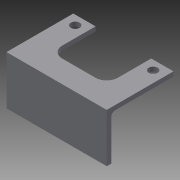
# Autodesk Inventor part: stpper holder
Saved by Autodesk Inventor 2015 (Build 190159000, 159)
## iProperties
Created: 2016-05-27
Part Number: stpper holder
Material: Generic
Document SubType Name: Modeling
Designer: Toby
Density: 1 g/cm^3
Appearance: Default
Author: Toby
Autodesk Inventor part; units mm, degrees
ref_plane "YZ Plane" through (0, 0, 0) normal (1, 0, 0) x (0, 1, 0)
ref_plane "XZ Plane" through (0, 0, 0) normal (0, 1, 0) x (-1, 0, 0)
ref_plane "XY Plane" through (0, 0, 0) normal (0, 0, 1) x (1, 0, 0)
sketch "Sketch1" plane through (0, 0, 0) normal (0, 0, 1) x (1, 0, 0)
  line L0 (-28.7318, -0.5685) -> (-18.7318, -0.5685)
  line L1 (-18.7318, -0.5685) -> (-18.7318, -30.5685)
  line L2 (-18.7318, -30.5685) -> (-28.7318, -30.5685)
  line L3 (-28.7318, -30.5685) -> (-28.7318, -0.5685)
  line L4 (-28.7318, -30.5685) -> (16.2682, -30.5685)
  line L5 (16.2682, -30.5685) -> (16.2682, -20.5685)
  line L6 (16.2682, -20.5685) -> (-28.7318, -20.5685)
  line L7 (-28.7318, -20.5685) -> (-28.7318, -30.5685)
  line L8 (16.2682, -30.5685) -> (6.2682, -30.5685)
  line L9 (6.2682, -30.5685) -> (6.2682, -0.5685)
  line L10 (6.2682, -0.5685) -> (16.2682, -0.5685)
  line L11 (16.2682, -0.5685) -> (16.2682, -30.5685)
  circle A0 centre (-23.7318, -4.6959) radius 2
  circle A1 centre (11.2682, -4.6959) radius 2
  point P0 (0, 0)
  dimension "d0" = 45
  dimension "d1" = 10
  dimension "d2" = 10
  dimension "d3" = 10
  dimension "d4" = 30
  dimension "d5" = 4
  dimension "d6" = 4
  constraints: 24 end point, 6 parallel, 3 horizontal, 3 perpendicular, 2 centre point, 1 point on line
  measures "d0" distance of L2.end L4.end
  measures "d1" distance of L0.start L0.end
  measures "d2" distance of L9.end L10.end
  measures "d3" distance between parallel lines of L4 L6
  measures "d4" distance of L2.end L0.start
  measures "d5" diameter of A0
  measures "d6" diameter of A1
extrude "Extrusion1" add sketch "Sketch1" along normal blind 2
fillet "Fillet1" radius 5 2 edges at (-18.7318, -20.5685, 1) (6.2682, -20.5685, 1)
sketch "Sketch2" plane through (0, 0, 0) normal (0, 0, -1) x (-1, 0, 0)
  line L0 (28.7318, -0.5685) -> (28.7318, -30.5685) projected
  line L1 (-16.1665, -30.4376) -> (28.7318, -30.4376)
  line L2 (28.7318, -30.4376) -> (28.7318, -28.4376)
  line L3 (28.7318, -28.4376) -> (-16.1665, -28.4376)
  line L4 (-16.1665, -28.4376) -> (-16.1665, -30.4376)
  point P0 (0, 0)
  dimension "d10" = 2
  constraints: 8 end point, 2 parallel, 1 horizontal, 1 perpendicular, 1 point on line
  measures "d10" distance between parallel lines of L3 L1
extrude "Extrusion2" add sketch "Sketch2" along normal blind 20
fillet "Fillet2" radius 2 1 edges at (-6.2826, -28.4376, 0)
body "Solid1"
